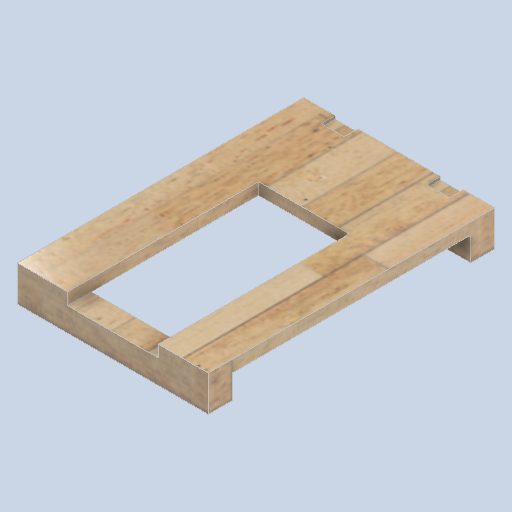
# Autodesk Inventor part: Part4
Saved by Autodesk Inventor 2022 (Build 260153000, 153)
## iProperties
Created: 2022-04-11
Part Number: Part4
Material: Wood (Maple)
Document SubType Name: Modeling
Designer: MacBook
Density: 0.67 g/cm^3
Appearance: Natural Maple - Glossy Dark Tint
Author: MacBook
Autodesk Inventor part; units mm, degrees
ref_plane "YZ Plane" through (0, 0, 0) normal (1, 0, 0) x (0, 1, 0)
ref_plane "XZ Plane" through (0, 0, 0) normal (0, 1, 0) x (-1, 0, 0)
ref_plane "XY Plane" through (0, 0, 0) normal (0, 0, 1) x (1, 0, 0)
sketch "Sketch1" plane through (0, 0, 0) normal (0, 1, 0) x (-1, 0, 0)
  line L0 (-152.4, -228.6) -> (152.4, -228.6)
  line L1 (152.4, -228.6) -> (152.4, 228.6)
  line L2 (152.4, 228.6) -> (-152.4, 228.6)
  line L3 (-152.4, 228.6) -> (-152.4, -228.6)
  line L4 (-152.4, -228.6) -> (152.4, 228.6) construction
  line L5 (152.4, -228.6) -> (-152.4, 228.6) construction
  point P0 (0, 0)
  dimension "d0" = 457.2
  dimension "d1" = 304.8
  constraints: 12 end point, 2 midpoint, 2 parallel, 1 horizontal, 1 perpendicular
  measures "d0" distance between parallel lines of L0 L2
  measures "d1" distance between parallel lines of L3 L1
extrude "Extrusion1" add sketch "Sketch1" against normal blind 19.05
sketch "Sketch3" plane through (0, -19.05, 0) normal (0, -1, 0) x (1, 0, 0)
  line L0 (152.4, -228.6) -> (152.4, 228.6) projected
  line L1 (-152.4, 228.6) -> (-152.4, -228.6) projected
  line L2 (152.4, 228.6) -> (-152.4, 228.6)
  line L3 (-152.4, 228.6) -> (-152.4, 190.5)
  line L4 (-152.4, 190.5) -> (152.4, 190.5)
  line L5 (152.4, 190.5) -> (152.4, 228.6)
  line L6 (-152.4, -228.6) -> (152.4, -228.6) projected
  line L7 (152.4, -190.5) -> (-152.4, -190.5)
  line L8 (-152.4, -190.5) -> (-152.4, -228.6)
  line L9 (-152.4, -228.6) -> (152.4, -228.6)
  line L10 (152.4, -228.6) -> (152.4, -190.5)
  point P0 (0, 0)
  dimension "d4" = 38.1
  dimension "d5" = 38.1
  constraints: 16 end point, 4 parallel, 2 horizontal, 2 perpendicular, 2 point on line
  measures "d4" distance between parallel lines of L2 L4
  measures "d5" distance between parallel lines of L6 L7
extrude "Extrusion2" add sketch "Sketch3" along normal blind 38.1 contours L6 L1 L7 L0 | L4 L1 L2 L0
sketch "Sketch4" plane through (0, 0, 0) normal (0, 1, 0) x (1, 0, 0)
  line L0 (-152.4, -228.6) -> (152.4, -228.6) projected
  line L1 (-72.2315, -228.6) -> (72.2315, -228.6)
  line L2 (72.2315, -228.6) -> (72.2315, 76.2)
  line L3 (72.2315, 76.2) -> (-72.2315, 76.2)
  line L4 (-72.2315, 76.2) -> (-72.2315, -228.6)
  line L5 (-152.4, 228.6) -> (-152.4, -228.6) projected
  point P0 (0, 0)
  dimension "d8" = 144.463
  dimension "d9" = 304.8
  dimension "d10" = 80.1685
  constraints: 8 end point, 2 parallel, 1 horizontal, 1 perpendicular, 1 point on line
  measures "d8" distance between parallel lines of L2 L4
  measures "d9" distance of L3.end L1.start
  measures "d10" distance between parallel lines of L5 L4
extrude "Extrusion3" cut sketch "Sketch4" against normal blind 19.05
sketch "Sketch5" plane through (0, 0, 0) normal (0, 1, 0) x (1, 0, 0)
  line L0 (-102.4, 228.6) -> (-65.887, 228.6)
  line L1 (-65.887, 228.6) -> (-65.887, 206.6)
  line L2 (-65.887, 206.6) -> (-102.4, 206.6)
  line L3 (-102.4, 206.6) -> (-102.4, 228.6)
  line L4 (152.4, 228.6) -> (-152.4, 228.6) projected
  line L5 (65.887, 228.6) -> (102.4, 228.6)
  line L6 (102.4, 228.6) -> (102.4, 206.6)
  line L7 (102.4, 206.6) -> (65.887, 206.6)
  line L8 (65.887, 206.6) -> (65.887, 228.6)
  line L9 (-152.4, 228.6) -> (-152.4, -228.6) projected
  line L10 (152.4, -228.6) -> (152.4, 228.6) projected
  point P0 (0, 0)
  point P1 (-65.887, 217.6)
  point P2 (84.1435, 228.6)
  dimension "d13" = 0
  dimension "d14" = 36.513
  dimension "d15" = 22
  dimension "d16" = 36.513
  dimension "d17" = 22
  dimension "d18" = 50
  dimension "d19" = 50
  constraints: 16 end point, 4 parallel, 2 horizontal, 2 midpoint, 2 perpendicular, 1 point on line
  measures "d13" distance between parallel lines of L4 L0
  measures "d14" distance from line of point (-65.887, 217.6) L3
  measures "d15" distance between parallel lines of L0 L2
  measures "d16" distance between parallel lines of L6 L8
  measures "d17" distance from line of point (84.144, 228.6) L7
  measures "d18" distance between parallel lines of L9 L3
  measures "d19" distance between parallel lines of L10 L6
extrude "Extrusion4" cut sketch "Sketch5" against normal blind 5
body "Solid1"
